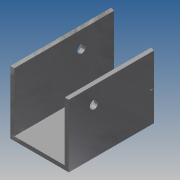
# Autodesk Inventor part: endChannelB
Saved by Autodesk Inventor 2014 SP1 (Build 180222100, 222)
## iProperties
Created: 2014-08-18
Part Number: endChannelB
Material: Steel, Galvanized
Document SubType Name: Modeling
Designer: Dave
Density: 7.85 g/cm^3
Appearance: Galvanized
Mass: 222.27 g
Surface Area: 199.608 cm^2
Volume: 28.3147 cm^3
d0: 1.500 in
d1: 1.750 in
d2: 1.750 in
d3: 0.120 in
d4: 3.000 in
d5: 0.00 deg
d6: 2.000 in
d7: 15.00 deg
d8: 4.000 in
d9: 0.00 deg
d10: 0.750 in
d11: 0.500 in
d12: 0.250 in
d17: 1.000 in
d18: 118.00 deg
d19: 2.000 in
d20: 0.500 in
d21: 0.250 in
d26: 1.000 in
d27: 118.00 deg
d28: 90.00 deg
d29: 0.100 in
d30: 0.100 in
d31: 4.000 in
d32: 0.00 deg
Author: Dave
Autodesk Inventor part; units mm, degrees
ref_plane "YZ Plane" through (0, 0, 0) normal (1, 0, 0) x (0, 1, 0)
ref_plane "XZ Plane" through (0, 0, 0) normal (0, 1, 0) x (-1, 0, 0)
sketch "Sketch1" plane through (0, 0, 0) normal (0, 0, 1) x (1, 0, 0)
  line L0 (0, 0) -> (38.1, 0)
  line L1 (38.1, 0) -> (38.1, 44.45)
  line L2 (0, 0) -> (0, 44.45)
  line L3 (-3.048, 44.45) -> (-3.048, -3.048)
  line L4 (-3.048, -3.048) -> (41.148, -3.048)
  line L5 (41.148, -3.048) -> (41.148, 44.45)
  line L6 (-3.048, 44.45) -> (0, 44.45)
  line L7 (38.1, 44.45) -> (41.148, 44.45)
  dimension "d0" = 38.1
  dimension "d1" = 44.45
  dimension "d2" = 44.45
  dimension "d3" = 3.048
  constraints: 16 end point, 3 equal length, 3 perpendicular, 1 horizontal, 2 other
  measures "d0" distance of L0.start L0.end
  measures "d1" distance of L0.end L1.end
  measures "d2" distance of L0.start L2.end
  measures "d3" distance between parallel lines of L3 L2
extrude "channel" add sketch "Sketch1" along normal blind 76.2
sketch "Sketch2" plane through (-3.048, 44.45, 0) normal (0, 1, 0) x (1, 0, 0)
  line L0 (0, 0) -> (49.069, -13.148)
  line L1 (0, 0) -> (50.8, 0) construction
  line L2 (0, 0) -> (49.069, 0)
  line L3 (49.069, -13.148) -> (49.069, 0)
  dimension "d6" = 50.8
  dimension "d7" = 15
  constraints: 8 end point, 1 equal length, 1 horizontal, 1 perpendicular
  measures "d6" distance of L0.start L0.end
  measures "d7" angle of L0 L1
extrude "angleCut" cut sketch "Sketch2" against normal blind 101.6
sketch "Sketch3" plane through (41.148, -3.048, 76.2) normal (1, 0, 0) x (0, 0, -1)
  line L0 (64.3577, 47.498) -> (0, 47.498) projected
  line L1 (0, 0) -> (0, 47.498) projected
  circle A0 centre (19.05, 34.798) radius 1.7319
  point P0 (76.2, 3.048)
  dimension "d10" = 19.05
  dimension "d11" = 12.7
  constraints: 1 centre point
  measures "d10" distance from line of A0.centre L1
  measures "d11" distance from line of A0.centre L0
hole "Hole1" at (41.148, 31.75, 57.15) direction (-1, 0, 0) diameter 6.35 depth 25.4 tip angle 118
sketch "Sketch5" plane through (-3.048, -3.048, 76.2) normal (-1, 0, 0) x (0, 0, 1)
  line L0 (0, 47.498) -> (0, 0) projected
  line L1 (-76.2, 47.498) -> (0, 47.498) projected
  circle A0 centre (-50.8, 34.798) radius 3.8194
  point P0 (-76.2, 3.048)
  dimension "d19" = 50.8
  dimension "d20" = 12.7
  constraints: 1 centre point
  measures "d19" distance from line of A0.centre L0
  measures "d20" distance from line of A0.centre L1
hole "Hole2" at (-3.048, 31.75, 25.4) direction (1, 0, 0) diameter 6.35 depth 25.4 tip angle 118
ref_plane "Work Plane1" through (41.148, 20.701, 11.8423) normal (-0.9659, 0, -0.2588) x (0, 1, 0)
sketch "Sketch6" plane through (41.148, 20.701, 11.8423) normal (-0.9659, 0, -0.2588) x (0, 1, 0)
  line L0 (1.5352, -0.3226) -> (-1.0048, -0.3226)
  line L1 (-1.0048, -0.3226) -> (-1.0048, -2.8626)
  line L2 (-1.0048, -2.8626) -> (1.5352, -2.8626)
  line L3 (1.5352, -2.8626) -> (1.5352, -0.3226)
  point P0 (-20.701, 0.7889)
  dimension "d29" = 2.54
  dimension "d30" = 2.54
  constraints: 8 end point, 2 parallel, 1 horizontal, 1 perpendicular
  measures "d29" distance of L2.end L1.end
  measures "d30" distance of L1.end L0.end
extrude "indentMark" cut sketch "Sketch6" against normal blind 101.6
body "Solid1"
